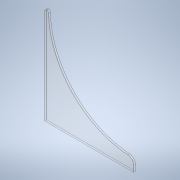
# Autodesk Inventor part: IndexCurveRail
Saved by Autodesk Inventor 2022 (Build 260153000, 153)
## iProperties
Created: 2022-01-14
Part Number: IndexCurveRail
Material: Polycarbonate, Clear
Document SubType Name: Modeling
Designer: tagaz
Density: 1.2 g/cm^3
Appearance: Polycarbonate - Clear
Author: tagaz
Autodesk Inventor part; units mm, degrees
ref_plane "YZ Plane" through (0, 0, 0) normal (1, 0, 0) x (0, 1, 0)
ref_plane "XZ Plane" through (0, 0, 0) normal (0, 1, 0) x (-1, 0, 0)
ref_plane "XY Plane" through (0, 0, 0) normal (0, 0, 1) x (1, 0, 0)
sketch "Sketch1" plane through (0, 0, 0) normal (0, 0, 1) x (1, 0, 0)
  arc A0 (-38.1, 0) -> (0, -38.1) centre (0, 0) ccw
  arc A1 (-266.6279, -6.2023) -> (-17.78, -266.1067) centre (0, 0) ccw
  line L0 (-272.9762, 0) -> (-273.05, 0)
  line L1 (0, -285.1143) -> (0, -304.8)
  line L2 (0, -304.8) -> (-279.4, -304.8)
  line L3 (-279.4, -304.8) -> (-279.4, -6.35)
  arc A2 (-273.05, 0) -> (-279.4, -6.35) centre (-273.05, -6.35) ccw
  arc A3 (-266.6279, -6.2023) -> (-272.9762, 0) centre (-272.9762, -6.35) ccw
  arc A4 (0, -285.1143) -> (-17.78, -266.1067) centre (-19.05, -285.1143) ccw
  point P0 (-266.7, 0)
  point P1 (0, -266.7)
  point P2 (-279.4, 0)
  dimension "d0" = 76.2
  dimension "d21" = 228.6
  dimension "d23" = 38.1
  dimension "d24" = 304.8
  dimension "d25" = 279.4
  dimension "d26" = 12.7
  dimension "d27" = 6.35
  dimension "d28" = 19.05
  constraints: 12 point on circle, 8 end point, 6 tangent, 5 centre point, 4 point on line, 3 perpendicular, 1 coincident, 1 equal radius, 1 horizontal
  measures "d0" diameter of A0
  measures "d21" radial gap between concentric circles of A0 A1
  measures "d23" distance of point (0, -266.7) L1.end
  measures "d24" distance from line of point (0, 0) L2
  measures "d25" distance from line of point (0, 0) L3
  measures "d26" distance of point (-266.7, 0) point (-279.4, 0)
  measures "d27" radius of A2
  measures "d28" radius of A4
extrude "Extrusion1" add sketch "Sketch1" along normal blind 6.35
fillet "Fillet3" radius 0.635 14 edges at (-268.5385, -1.808, 6.35) (-273.0131, 0, 6.35) (-277.5401, -1.8599, 6.35) (-279.4, -155.575, 6.35) (-5.1378, -272.1007, 6.35) (0, -294.9571, 6.35) (-192.6383, -184.4434, 6.35) (-268.5385, -1.808, 0) (-273.0131, 0, 0) (-277.5401, -1.8599, 0) (-279.4, -155.575, 0) (-5.1378, -272.1007, 0) (0, -294.9571, 0) (-192.6383, -184.4434, 0)
body "Solid1"
